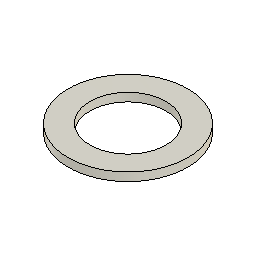
Spacing Washer v2 (Autodesk Fusion 360 design; units mm, degrees)
Autodesk Fusion 360 part; units mm, degrees
sketch "Sketch1" plane through (0, 0, 0) normal (0, 0, 1) x (1, 0, 0)
  circle A0 centre (0, 0) radius 23.1775
  circle A1 centre (0, 0) radius 36.576
  dimension "d1" = 46.355
  dimension "d2" = 73.152
  constraint coincident A0.centre A1.centre
  measures "d1" diameter of A0
  measures "d2" diameter of A1
extrude "Extrude1" add sketch "Sketch1" along normal blind 5.08
equation "d3 = 2.54 * 2 mm"
